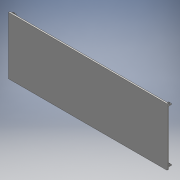
# Autodesk Inventor part: Bumper big
Saved by Autodesk Inventor 2016 (Build 200138000, 138)
## iProperties
Created: 2016-10-11
Part Number: Bumper big
Material: Generic
Document SubType Name: Modeling
Designer: yurra
Density: 1 g/cm^3
Appearance: Default
Author: yurra
Autodesk Inventor part; units mm, degrees
ref_plane "YZ Plane" through (0, 0, 0) normal (1, 0, 0) x (0, 1, 0)
ref_plane "XZ Plane" through (0, 0, 0) normal (0, 1, 0) x (-1, 0, 0)
ref_plane "XY Plane" through (0, 0, 0) normal (0, 0, 1) x (1, 0, 0)
sketch "Sketch1" plane through (0, 0, 0) normal (0, 1, 0) x (-1, 0, 0)
  line L0 (89.45, 32.5) -> (-89.45, 32.5)
  line L1 (-89.45, 32.5) -> (-89.45, -32.5)
  line L2 (-89.45, -32.5) -> (89.45, -32.5)
  line L3 (89.45, -32.5) -> (89.45, 32.5)
  line L4 (89.45, 32.5) -> (-89.45, -32.5) construction
  line L5 (-89.45, 32.5) -> (89.45, -32.5) construction
  point P0 (0, 0)
  dimension "d0" = 178.9
  dimension "d1" = 65
  constraints: 12 end point, 2 midpoint, 2 parallel, 1 horizontal, 1 perpendicular
  measures "d0" distance of L2.end L1.end
  measures "d1" distance of L1.end L0.end
extrude "Extrusion1" add sketch "Sketch1" along normal blind 1.5
sketch "Sketch2" plane through (0, 1.5, 0) normal (0, 1, 0) x (1, 0, 0)
  line L0 (89.45, -32.5) -> (89.45, 32.5) projected
  line L1 (-89.45, -29.75) -> (89.45, -29.75)
  line L2 (89.45, -29.75) -> (89.45, 29.75)
  line L3 (89.45, 29.75) -> (-89.45, 29.75)
  line L4 (-89.45, 29.75) -> (-89.45, -29.75)
  line L5 (-89.45, -29.75) -> (89.45, 29.75) construction
  line L6 (89.45, -29.75) -> (-89.45, 29.75) construction
  line L7 (89.45, 29.75) -> (85.95, 29.75)
  line L8 (85.95, 29.75) -> (85.95, 30.25)
  line L9 (85.95, 30.25) -> (89.45, 30.25)
  line L10 (89.45, 30.25) -> (89.45, 29.75)
  line L11 (85.95, 29.75) -> (85.95, 29.25)
  line L12 (85.95, 29.25) -> (89.45, 29.25)
  line L13 (89.45, 29.25) -> (89.45, 29.75)
  line L14 (0, 0) -> (0, 29.75)
  line L15 (0, 0) -> (37, 0)
  line L16 (-89.45, 29.75) -> (-85.95, 29.75)
  line L17 (-85.95, 29.75) -> (-85.95, 30.25)
  line L18 (-85.95, 30.25) -> (-89.45, 30.25)
  line L19 (-89.45, 30.25) -> (-89.45, 29.75)
  line L20 (-85.95, 29.75) -> (-85.95, 29.25)
  line L21 (-85.95, 29.25) -> (-89.45, 29.25)
  line L22 (-89.45, 29.25) -> (-89.45, 29.75)
  line L23 (89.45, -29.75) -> (85.95, -29.75)
  line L24 (85.95, -29.75) -> (85.95, -30.25)
  line L25 (85.95, -30.25) -> (89.45, -30.25)
  line L26 (89.45, -30.25) -> (89.45, -29.75)
  line L27 (85.95, -29.75) -> (85.95, -29.25)
  line L28 (85.95, -29.25) -> (89.45, -29.25)
  line L29 (89.45, -29.25) -> (89.45, -29.75)
  line L30 (-89.45, -29.75) -> (-85.95, -29.75)
  line L31 (-85.95, -29.75) -> (-85.95, -30.25)
  line L32 (-89.45, -30.25) -> (-89.45, -29.75)
  line L33 (-85.95, -29.75) -> (-85.95, -29.25)
  line L34 (-85.95, -29.25) -> (-89.45, -29.25)
  line L35 (-89.45, -29.25) -> (-89.45, -29.75)
  line L36 (-85.95, -30.25) -> (-89.45, -30.25)
  dimension "d4" = 59.5
  dimension "d5" = 3.5
  dimension "d6" = 0.5
  constraints: 72 end point, 17 symmetric about line, 4 parallel, 3 midpoint, 2 horizontal, 2 perpendicular, 2 point on line
  measures "d4" distance of L2.end L1.end
  measures "d5" distance of L2.end L7.end
  measures "d6" distance of L7.end L8.end
extrude "Extrusion2" add sketch "Sketch2" along normal blind 3.5 contours L25 L24 L1 L0 | L1 L27 L28 L0 | L12 L11 L3 L0 | L31 L36 L32 L1 | L1 L4 L34 L33 | L3 L8 L9 L0 | L4 L3 L20 L21 | L3 L19 L18 L17
hole "Hole1" at (-87.7, 3.25, 30.25) direction (0, 0, -1) diameter 3 end through all
hole "Hole2" at (87.7, 3.25, 30.25) direction (0, 0, -1) diameter 3 end through all
body "Solid1"
